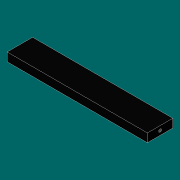
# Autodesk Inventor part: detectorSuppourt
Saved by Autodesk Inventor 2016 SP1 (Build 200210100, 210)
## iProperties
Created: 2015-10-27
Part Number: detectorSuppourt
Material: ABS Plastic
Document SubType Name: Modeling
Designer: Sawaiz
Density: 1.06 g/cm^3
Appearance: Smooth - Black
Author: Sawaiz
Autodesk Inventor part; units mm, degrees
ref_plane "YZ Plane" through (0, 0, 0) normal (1, 0, 0) x (0, 1, 0)
ref_plane "XZ Plane" through (0, 0, 0) normal (0, 1, 0) x (-1, 0, 0)
ref_plane "XY Plane" through (0, 0, 0) normal (0, 0, 1) x (1, 0, 0)
sketch "Sketch1" plane through (0, 0, 0) normal (0, 0, 1) x (1, 0, 0)
  line L0 (-9.525, -52.5) -> (9.525, -52.5)
  line L1 (9.525, -52.5) -> (9.525, 52.5)
  line L2 (9.525, 52.5) -> (-9.525, 52.5)
  line L3 (-9.525, 52.5) -> (-9.525, -52.5)
  line L4 (-9.525, -52.5) -> (9.525, 52.5) construction
  line L5 (9.525, -52.5) -> (-9.525, 52.5) construction
  point P0 (0, 0)
  dimension "d0" = 19.05
  dimension "d1" = 105
  constraints: 12 end point, 2 midpoint, 2 parallel, 1 horizontal, 1 perpendicular
  measures "d0" distance of L2.end L1.end
  measures "d1" distance of L1.end L0.end
extrude "Extrusion1" add sketch "Sketch1" along normal blind 6.35
sketch "Sketch3" plane through (-9.525, 52.5, 0) normal (0, 1, 0) x (1, 0, 0)
  line L0 (19.05, 0) -> (0, 0) projected
  line L1 (0, 0) -> (0, -6.35) projected
  line L2 (19.05, -6.35) -> (0, -6.35) projected
  line L3 (19.05, 0) -> (19.05, -6.35) projected
  line L4 (0, 0) -> (0, -6.35) projected
  line L5 (0, 0) -> (19.05, -6.35)
  point P0 (9.525, 0)
  point P1 (9.525, -3.175)
  constraints: 2 end point, 1 midpoint
hole "Hole1" at (0, 52.5, 3.175) direction (0, -1, 0) diameter 2.156 depth 8.865 tip angle 118 thread size "4-40 UNC" class "2B" standard "ANSI Unified Screw Threads"
mirror "Mirror1" about plane through (0, 0, 0) normal (0, 1, 0) of "Hole1"
equation "\"d0\" = sensorHolderDepth"
equation "\"d2\" = acrylicThickness"
equation "\"acrylicThickness\" = 6.35"
equation "\"height\" = 127"
equation "\"width\" = 127"
equation "\"depth\" = 273.05"
equation "\"mirrorAngle\" = 5deg"
equation "\"detectorWidth\" = 52"
equation "\"detectorHeight\" = 52"
equation "\"mirrorThickness\" = 3.175"
equation "\"fresnelThickness\" = 0.1"
equation "\"focalLength\" = 76.2"
equation "\"ior\" = 1.49"
equation "\"centerThickness\" = 1.524"
equation "\"fresnelAngle\" = 90deg"
equation "\"fresnelEffectiveDiameter\" = 152.4"
equation "\"mirrorSuppourtWidth\" = 38.1"
equation "\"backGrooveBit\" = 4.8006"
equation "\"detectorOpeningWidth\" = 76.2"
equation "\"detectorOpeningHeight\" = 76.2"
equation "\"sensorHolderSensorHeight\" = 53.975"
equation "\"sensorHolderSensorWidth\" = 53.975"
equation "\"oRingWidth\" = 1.5875"
equation "\"sensorHolderORingID\" = 203.2"
equation "\"sensorHolderFlushORingID\" = 304.8"
equation "\"frontBackORingID\" = 419.1"
equation "\"mirrorGroove\" = 19.05"
equation "\"backMirrorGroove\" = 6.35"
equation "\"fresnelMirrorChamfer\" = 6.35"
equation "\"mirrorGrooveMill\" = 3.175"
equation "\"sensorHolderDepth\" = 19.05"
equation "\"frameAcrylicThickness\" = 9.525"
equation "\"internalAcrylicThicnkess\" = 6.35"
equation "\"internalAcrylicThickness\" = 6.35"
equation "\"aerogelClearence\" = 3.175"
equation "\"backplanePCBWidth\" = 76.2"
equation "\"backplanePostionOffsett\" = 12.7"
equation "\"backplaneHoleOffsett\" = 6.35"
equation "\"backplanePCBHeight\" = 76.2"
equation "\"moduleSlotClearence\" = 0.79375"
body "Solid1"
